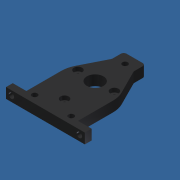
# Autodesk Inventor part: EllbowMotorMount
Saved by Autodesk Inventor 2014 SP2 (Build 180246200, 246)
## iProperties
Created: 2015-02-01
Part Number: EllbowMotorMount
Material: ABS-Kunststoff - Schwarz
Document SubType Name: Modeling
Designer: 4ndreas
Density: 1.06 g/cm^3
Appearance: Glatt - weiß(2)
Author: 4ndreas
Autodesk Inventor part; units mm, degrees
ref_plane "YZ Plane" through (0, 0, 0) normal (1, 0, 0) x (0, 1, 0)
ref_plane "XZ Plane" through (0, 0, 0) normal (0, 1, 0) x (-1, 0, 0)
ref_plane "XY Plane" through (0, 0, 0) normal (0, 0, 1) x (1, 0, 0)
sketch "Skizze1" plane through (0, 0, 0) normal (0, 0, 1) x (1, 0, 0)
  arc A0 (-19, -51.1238) -> (19, -51.1238) centre (0, -51.1238) ccw projected
  line L0 (-19, -72.2231) -> (-19, -51.1238) projected
  line L1 (-19, -72.2231) -> (-29, -72.2231) projected
  line L2 (-29, -72.2231) -> (-29, -77.2231) projected
  line L3 (29, -77.2231) -> (-29, -77.2231) projected
  line L4 (29, -77.2231) -> (29, -72.2231) projected
  line L5 (29, -72.2231) -> (19, -72.2231) projected
  line L6 (19, -72.2231) -> (19, -51.1238) projected
  circle A1 centre (0, -47.6238) radius 17.5 projected
  circle A2 centre (0, -40.6238) radius 6 projected
  arc A3 (19, -46.6238) -> (-19, -46.6238) centre (0, -46.6238) ccw
  line L7 (-19, -46.6238) -> (-19, -51.1238)
  line L8 (19, -46.6238) -> (19, -51.1238)
  circle A4 centre (-13.446, -71.669) radius 2.1 projected
  circle A5 centre (13.446, -71.669) radius 2.1 projected
  point P0 (0, 0)
  constraints: 4 end point, 2 collinear, 2 point on circle, 2 tangent, 1 centre point, 1 vertical alignment, 1 other
extrude "Extrusion1" add sketch "Skizze1" along normal blind 8 contours L7 A3 L8 A0 | A0 L6 L5 L4 L3 L2 L1 L0 | A1 | A4 | A5
sketch "Skizze2" plane through (-29, -77.2231, 0) normal (0, -1, 0) x (1, 0, 0)
  circle A0 centre (4, 4.5) radius 2.35 projected
  circle A1 centre (54, 4.5) radius 2.35 projected
  point P0 (29, 0)
hole "Bohrung1" at (-25, -77.2231, 4.5) at (25, -77.2231, 4.5) direction (0, 1, 0) diameter 4 end through all
sketch "Skizze3" plane through (0, 0, 0) normal (0, 0, -1) x (-1, 0, 0)
  circle A0 centre (0, -40.6238) radius 6 projected
  line L0 (-19, -72.2231) -> (-19, -46.6238) projected
  line L1 (-29, -72.2231) -> (-19, -72.2231) projected
  line L2 (-29, -77.2231) -> (-29, -72.2231) projected
  line L3 (29, -77.2231) -> (-29, -77.2231) projected
  line L4 (29, -72.2231) -> (29, -77.2231) projected
  line L5 (19, -72.2231) -> (29, -72.2231) projected
  line L6 (19, -46.6238) -> (19, -72.2231) projected
  arc A1 (19, -46.6238) -> (-19, -46.6238) centre (0, -46.6238) ccw projected
  point P0 (0, 0)
extrude "Extrusion2" cut sketch "Skizze3" against normal blind 0.5
sketch "Skizze4" plane through (0, 0, 8) normal (0, 0, 1) x (1, 0, 0)
  circle A0 centre (-13.446, -71.669) radius 2.1 projected
  circle A1 centre (13.446, -71.669) radius 2.1 projected
  point P0 (0, 0)
hole "Bohrung2" at (-13.446, -71.669, 8) at (13.446, -71.669, 8) direction (0, 0, -1) diameter 4 end through all
sketch "Skizze5" plane through (0, 0, 0.5) normal (0, 0, -1) x (-1, 0, 0)
  circle A0 centre (13.446, -71.669) radius 2 projected
  circle A1 centre (-13.446, -71.669) radius 2 projected
  line L0 (-19, -72.2231) -> (-19, -46.6238) projected
  line L1 (19, -46.6238) -> (19, -72.2231) projected
  line L2 (-13.446, -67.6276) -> (-9.946, -69.6483)
  line L3 (-9.946, -69.6483) -> (-9.946, -73.6898)
  line L4 (-9.946, -73.6898) -> (-13.446, -75.7105)
  line L5 (-13.446, -75.7105) -> (-16.946, -73.6898)
  line L6 (-16.946, -73.6898) -> (-16.946, -69.6483)
  line L7 (-16.946, -69.6483) -> (-13.446, -67.6276)
  line L8 (13.446, -67.6276) -> (16.946, -69.6483)
  line L9 (16.946, -69.6483) -> (16.946, -73.6898)
  line L10 (16.946, -73.6898) -> (13.446, -75.7105)
  line L11 (13.446, -75.7105) -> (9.946, -73.6898)
  line L12 (9.946, -73.6898) -> (9.946, -69.6483)
  line L13 (9.946, -69.6483) -> (13.446, -67.6276)
  point P0 (0, 0)
  dimension "d18" = 7
  constraints: 24 end point, 3 parallel, 2 coincident, 26 other
  measures "d18" distance between parallel lines of L6 L3
extrude "Extrusion3" cut sketch "Skizze5" against normal blind 3 contours A0 | A1 | L2 L3 L4 L5 L6 L7 | L8 L9 L10 L11 L12 L13
sketch "Skizze8" plane through (0, 0, 8) normal (0, 0, 1) x (1, 0, 0)
  circle A0 centre (0, -40.6238) radius 6 projected
  line L0 (-29, -77.2231) -> (29, -77.2231) projected
  circle A1 centre (0, -47.6238) radius 15.5 construction
  line L1 (0, -40.6238) -> (0, -77.2231) construction
  line L2 (-13.4234, -39.8738) -> (0, -47.6238) construction
  line L3 (0, -47.6238) -> (13.4234, -39.8738) construction
  line L4 (0, -47.6238) -> (0, -32.1238) construction
  point P0 (0, 0)
  point P1 (0, -63.1238)
  dimension "d21" = 31
  dimension "d22" = 7
  dimension "d23" = 60
  constraints: 8 end point, 4 point on circle, 2 coincident, 2 point on line, 1 centre point, 1 collinear, 1 midpoint, 1 other
  measures "d21" diameter of A1
  measures "d22" distance of L2.end L1.start
  measures "d23" angle of L3 L4
hole "Bohrung3" at (-13.4234, -39.8738, 8) at (13.4234, -39.8738, 8) at (0, -63.1238, 8) direction (0, 0, -1) diameter 3.2 end through all counterbore diameter 6 counterbore depth 3
sketch "Skizze9" plane through (0, 0, 8) normal (0, 0, 1) x (1, 0, 0)
  circle A0 centre (0, -40.6238) radius 6 projected
  circle A1 centre (0, -40.6238) radius 6.1
  point P0 (0, 0)
  dimension "d31" = 12.2
  constraints: 1 centre point
  measures "d31" diameter of A1
extrude "Extrusion4" cut sketch "Skizze9" against normal through all contours A0 | A1
sketch "Skizze10" plane through (0, 0, 3.5) normal (0, 0, -1) x (-1, 0, 0)
  circle A0 centre (13.446, -71.669) radius 2 projected
  circle A1 centre (-13.446, -71.669) radius 2 projected
  circle A2 centre (-13.446, -71.669) radius 2 projected
  line L0 (-13.446, -67.6276) -> (-9.946, -69.6483) projected
  line L1 (-16.946, -69.6483) -> (-13.446, -67.6276) projected
  line L2 (-16.946, -73.6898) -> (-16.946, -69.6483) projected
  line L3 (-13.446, -75.7105) -> (-16.946, -73.6898) projected
  line L4 (-9.946, -73.6898) -> (-13.446, -75.7105) projected
  line L5 (-9.946, -69.6483) -> (-9.946, -73.6898) projected
  point P0 (0, 0)
extrude "Extrusion5" add sketch "Skizze10" against normal blind 0.2 contours A0 | A1
sketch "Skizze11" plane through (0, 0, 8) normal (0, 0, 1) x (1, 0, 0)
  circle A0 centre (0, -63.1238) radius 3 projected
  arc A1 (19, -46.6238) -> (-19, -46.6238) centre (0, -46.6238) ccw projected
  arc A2 (15, -16.1238) -> (15, -21.1238) centre (15, -18.6238) ccw construction
  line L0 (15, -16.1238) -> (23, -16.1238) construction
  arc A3 (23, -21.1238) -> (23, -16.1238) centre (23, -18.6238) ccw construction
  line L1 (23, -21.1238) -> (15, -21.1238) construction
  arc A4 (-23, -16.1238) -> (-23, -21.1238) centre (-23, -18.6238) ccw construction
  line L2 (-23, -16.1238) -> (-15, -16.1238) construction
  arc A5 (-15, -21.1238) -> (-15, -16.1238) centre (-15, -18.6238) ccw construction
  line L3 (-15, -21.1238) -> (-23, -21.1238) construction
  line L4 (23, -25.6238) -> (-23, -25.6238) construction
  arc A6 (23, -25.6238) -> (23, -11.6238) centre (23, -18.6238) ccw construction
  line L5 (-23, -11.6238) -> (23, -11.6238) construction
  arc A7 (-23, -11.6238) -> (-23, -25.6238) centre (-23, -18.6238) ccw construction
  line L6 (-8, -29.3901) -> (8, -29.3901)
  line L7 (8, -29.3901) -> (8, -13.6238)
  line L8 (6, -11.6238) -> (-6, -11.6238)
  line L9 (-8, -13.6238) -> (-8, -29.3901)
  line L10 (0, -63.1238) -> (0, -11.6238) construction
  circle A8 centre (-15, -18.6238) radius 7 construction
  arc A9 (-6, -11.6238) -> (-8, -13.6238) centre (-6, -13.6238) ccw
  arc A10 (8, -13.6238) -> (6, -11.6238) centre (6, -13.6238) ccw
  line L11 (-8, -20.2888) -> (-16.9654, -38.0696)
  line L12 (8, -20.2888) -> (16.9654, -38.0696)
  circle A11 centre (0, -18.6238) radius 2 projected
  point P0 (0, 0)
  point P1 (8, -11.6238)
  dimension "d36" = 2
  constraints: 14 end point, 8 tangent, 7 point on circle, 5 point on line, 3 centre point, 2 parallel, 2 perpendicular, 1 coincident, 1 equal radius, 1 horizontal, 1 midpoint, 2 other
  measures "d36" radius of A9
extrude "Extrusion6" add sketch "Skizze11" against normal up to surface (7.5 mm away) contours A1 L7 L12 | A1 L9 A9 L8 A10 L7 | A1 L11 L9 | A11
fillet "Rundung1" radius 3 2 edges at (-8, -20.2888, 4.25) (8, -20.2888, 4.25)
sketch "Skizze12" plane through (0, 0, 0.5) normal (0, 0, -1) x (-1, 0, 0)
  circle A0 centre (0, -63.1238) radius 1.6 projected
  line L0 (6, -11.6238) -> (-6, -11.6238) projected
  line L1 (-8, -13.6238) -> (-8, -19.5752) projected
  arc A1 (-23, -16.1238) -> (-23, -21.1238) centre (-23, -18.6238) ccw projected
  arc A2 (23, -21.1238) -> (23, -16.1238) centre (23, -18.6238) ccw projected
  line L2 (-23, -18.6238) -> (23, -18.6238) construction
  line L3 (0, -11.6238) -> (0, -63.1238) construction
  point P0 (0, 0)
  point P1 (0, -18.6238)
  constraints: 4 end point, 2 midpoint, 2 perpendicular, 1 point on line
hole "Bohrung4" at (0, -18.6238, 0.5) direction (0, 0, 1) diameter 4 end through all
sketch "Skizze13" plane through (0, 0, 0.5) normal (0, 0, -1) x (-1, 0, 0)
  circle A0 centre (0, -18.6238) radius 2 projected
  line L0 (-8, -13.6238) -> (-8, -19.5752) projected
  line L1 (0, -14.5824) -> (3.5, -16.6031)
  line L2 (3.5, -16.6031) -> (3.5, -20.6446)
  line L3 (3.5, -20.6446) -> (0, -22.6653)
  line L4 (0, -22.6653) -> (-3.5, -20.6446)
  line L5 (-3.5, -20.6446) -> (-3.5, -16.6031)
  line L6 (-3.5, -16.6031) -> (0, -14.5824)
  point P0 (0, 0)
  dimension "d47" = 7
  constraints: 12 end point, 1 coincident, 1 parallel, 13 other
  measures "d47" distance between parallel lines of L2 L5
extrude "Extrusion7" cut sketch "Skizze13" against normal blind 3 contours A0 | L1 L2 L3 L4 L5 L6
sketch "Skizze14" plane through (0, 0, 3.5) normal (0, 0, -1) x (-1, 0, 0)
  circle A0 centre (0, -18.6238) radius 2 projected
  point P0 (0, 0)
extrude "Extrusion8" add sketch "Skizze14" against normal blind 0.2
